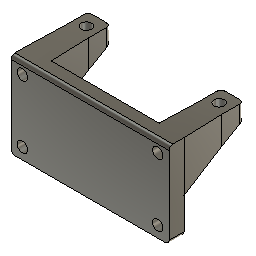
project (Autodesk Fusion 360 design; units mm, degrees)
Autodesk Fusion 360 part; units mm, degrees
sketch "Sketch1" plane through (0, 0, 0) normal (0, 1, 0) x (1, 0, 0)
  line L0 (-27, 29.5) -> (27, 29.5) construction
  line L1 (27, 29.5) -> (27, 4.5) construction
  line L2 (27, 4.5) -> (-27, 4.5) construction
  line L3 (-27, 4.5) -> (-27, 29.5) construction
  circle A0 centre (-27, 4.5) radius 2.085
  circle A1 centre (27, 4.5) radius 2.085
  circle A2 centre (27, 29.5) radius 2.085
  circle A3 centre (-27, 29.5) radius 2.085
  line L4 (-31.5, 34) -> (31.5, 34)
  line L5 (31.5, 34) -> (31.5, 0)
  line L6 (31.5, 0) -> (-31.5, 0)
  line L7 (-31.5, 0) -> (-31.5, 34)
  dimension "d1" = 4.17
  dimension "d2" = 54
  dimension "d3" = 25
  dimension "d4" = -4.5
  dimension "d14" = 34
  constraint horizontal L0
  constraint vertical L1
  constraint horizontal L2
  constraint vertical L3
  constraint coincident L2.end L3.start
  constraint coincident L1.end L2.start
  constraint coincident L0.end L1.start
  constraint coincident L0.start L3.end
  constraint equal A0 A1
  constraint equal A2 A3
  constraint equal A0 A3
  constraint midpoint origin L6
  measures "d1" diameter of A0
  measures "d2" distance of L1.end L2.end
  measures "d3" distance of L0.start L2.end
  measures "d14" distance of L4.end L5.end
sketch "Sketch2" plane through (0, 0, 0) normal (0, 0, 1) x (1, 0, 0)
  line L0 (-26.5, 25) -> (26.5, 25) construction
  line L1 (31.5, 0) -> (-31.5, 0)
  line L2 (0, 25) -> (0, 0) construction
  line L3 (-31.5, 0) -> (31.5, 0) construction
  circle A0 centre (-26.5, 25) radius 2.085
  line L4 (-31, 21.237) -> (-31, 30.237)
  line L5 (-31, 30.237) -> (-22, 30.237)
  line L6 (-22, 30.237) -> (-22, 21.237)
  line L7 (-22, 19.763) -> (-31, 30.237) construction
  line L8 (-31.5, 0) -> (-31.5, 6)
  line L9 (-31.5, 6) -> (-31, 21.237)
  line L10 (-26.5, 25) -> (-26.5, 0) construction
  line L11 (-21.5, 6) -> (-22, 21.237)
  line L12 (-21.5, 6) -> (0, 6)
  line L13 (31.5, 0) -> (31.5, 6)
  line L14 (31, 21.237) -> (31, 30.237)
  line L15 (31, 30.237) -> (22, 30.237)
  line L16 (22, 30.237) -> (22, 21.237)
  line L17 (31.5, 6) -> (31, 21.237)
  line L18 (21.5, 6) -> (0, 6)
  line L19 (21.5, 6) -> (22, 21.237)
  circle A1 centre (26.5, 25) radius 2.085
  dimension "d5" = 53
  dimension "d6" = 25
  dimension "d8" = 4.17
  dimension "d9" = 9
  dimension "d23" = 6
  dimension "d32" = 15.237
  constraint horizontal L0
  constraint midpoint L0 L2.start
  constraint coincident L2.end origin
  constraint vertical L2
  constraint coincident L0.start A0.centre
  constraint vertical L4
  constraint horizontal L5
  constraint vertical L6
  constraint midpoint L0.start L7
  constraint equal L5 L6
  constraint coincident L1.end L3.start
  constraint perpendicular L3 L8
  constraint coincident L1 L10.end
  constraint vertical L10
  constraint symmetric L4.start L10 L6.end
  constraint symmetric L8.end L10 L11.start
  constraint coincident L2 L12.end
  constraint horizontal L12
  constraint coincident L7.start L6
  constraint coincident L6.end L11.end
  constraint symmetric L2 A0 A1
  constraint symmetric L2 L4.start L14.start
  constraint symmetric L2 L4.end L14.end
  constraint symmetric L2 L5.end L15.end
  constraint symmetric L2 L1.end L1.start
  constraint symmetric L2 L8.end L13.end
  constraint symmetric L2 L11.start L18.start
  constraint symmetric L2 L6.end L16.end
  constraint symmetric L2 L12.end L18.end
  measures "d5" distance of L0.start L0.end
  measures "d6" distance of L0 L1
  measures "d8" diameter of A0
  measures "d9" distance of L4.end L5.end
  measures "d23" distance of L1.end L8.end
  measures "d32" vertical distance of L4.start L8.end
extrude "Extrude3" add sketch "Sketch1" along normal blind 6 contours A0 | A1 | A2 | A3 | L4 L5 L6 L7
extrude "Extrude4" add sketch "Sketch2" against normal blind 6 contours L1 L4 L5 L6 L8 L9 L11 L12 L13 L14 L15 L16 L17 L18 L19 | A0 | A1
extrude "Extrude5" cut sketch "Sketch1" along normal blind 4.5 contours A0 | A1 | A2 | A3
extrude "Extrude6" cut sketch "Sketch2" against normal blind 4.5 contours A0 | A1
fillet "Fillet4" radius 1.5 7 edges at (0, 0, 0) (31.5, 3, -34) (-31.5, 3, -34) (-22, 30.237, -3) (-31, 30.237, -3) (22, 30.237, -3) (31, 30.237, -3)
draft "Draft1" angle 30 neutral plane through (31, 30.237, 0) pull (0, 1, 0) 2 faces at (28, 11.079, -6) (-25, 11.079, -6)
equation "d1 = InsertWidth"
equation "InsertWidth = 4.17 mm"
equation "d8 = InsertWidth"
equation "InsertLength = 4.5 mm"
equation "Thickness = 6 mm"
equation "d19 = Thickness"
equation "d21 = -Thickness"
equation "d23 = Thickness"
equation "d24 = InsertLength"
equation "d26 = -InsertLength"
